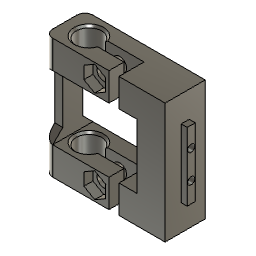
NAN dovetail rod mount - concept 2 v13 (Autodesk Fusion 360 design; units mm, degrees)
Autodesk Fusion 360 part; units mm, degrees
sketch "Sketch1" plane through (0, 0, 0) normal (0, 1, 0) x (1, 0, 0)
  line L0 (15, 15) -> (-15, 15)
  line L1 (-15, 15) -> (-15, -15)
  line L2 (-15, -15) -> (15, -15)
  line L3 (15, -15) -> (15, 15)
  line L4 (15, 15) -> (-15, -15) construction
  line L5 (-15, 15) -> (15, -15) construction
  dimension "d1" = 30
  dimension "d2" = 30
  constraint horizontal L0
  constraint perpendicular L0 L1
  constraint parallel L0 L2
  constraint parallel L1 L3
  constraint coincident L4 origin
  constraint coincident L5 origin
  measures "d1" distance of L1.end L2.end
  measures "d2" distance of L0.start L2.end
extrude "Extrude1" add sketch "Sketch1" along normal mid plane 10
sketch "Sketch2" plane through (0, 0, 15) normal (0, 0, 1) x (-1, 0, 0)
  line L0 (-15, 5) -> (-15, -5)
  line L1 (-15, -5) -> (15, -5)
  line L2 (15, -5) -> (15, 5)
  line L3 (15, 5) -> (-15, 5)
  point P0 (9, 0)
  dimension "d5" = 6
  measures "d5" distance of L2 P0
hole "Hole1" at (-9, 0, 15) direction (0, 0, -1) diameter 6.35 end through all
sketch "Sketch3" plane through (0, 0, 15) normal (0, 0, 1) x (-1, 0, 0)
  circle A0 centre (9, 0) radius 3.175
  line L0 (-15, 5) -> (-15, -5)
  line L1 (-15, -5) -> (15, -5)
  line L2 (15, -5) -> (15, 5)
  line L3 (15, 5) -> (-15, 5)
  line L4 (-3.5, -1.25) -> (11.5, -1.25)
  line L5 (11.5, -1.25) -> (11.5, 1.25)
  line L6 (11.5, 1.25) -> (-3.5, 1.25)
  line L7 (-3.5, 1.25) -> (-3.5, -1.25)
  line L8 (-3.5, -1.25) -> (11.5, 1.25) construction
  line L9 (11.5, -1.25) -> (-3.5, 1.25) construction
  line L10 (-3.5, 1.25) -> (-1, 1.25)
  line L11 (-1, 1.25) -> (-1, 5)
  line L12 (-3.5, 5) -> (-3.5, 1.25)
  point P0 (4, 0)
  dimension "d9" = 5
  dimension "d10" = 2.5
  dimension "d11" = 15
  dimension "d18" = 2.5
  constraint horizontal L4
  constraint perpendicular L4 L5
  constraint parallel L4 L6
  constraint parallel L5 L7
  constraint coincident L8 P0
  constraint coincident L9 P0
  constraint horizontal A0.centre P0
  constraint horizontal L10
  constraint vertical L11
  constraint vertical L12
  constraint coincident L3 L11.end
  constraint coincident L3 L12.start
  measures "d9" distance of A0.centre P0
  measures "d10" distance of L4.start L6.end
  measures "d11" distance of L5.end L6.end
  measures "d18" distance of L11 L12
extrude "Extrude2" cut sketch "Sketch3" against normal through all contours A0 L4 L6 L7 L10 | L3 L6 L10 L11 L12
sketch "Sketch4" plane through (0, 5, 0) normal (0, 1, 0) x (-1, 0, 0)
  line L0 (-15, 15) -> (-15, -15)
  line L1 (-15, -15) -> (15, -15)
  line L2 (15, -15) -> (15, 15)
  line L3 (15, 15) -> (-15, 15)
  line L4 (-1, -15) -> (6.0814, -15)
  line L5 (6.0814, -15) -> (6.0814, 15)
  line L6 (6.0814, 15) -> (-1, 15)
  line L7 (-1, 15) -> (-1, -15)
  point P0 (2.5407, 11.5)
  point P1 (2.5407, 15)
  dimension "d14" = 3.5
  constraint midpoint L6 P1
  constraint vertical P0 P1
  measures "d14" distance of P0 P1
hole "Hole2" at (-2.5407, 5, 11.5) direction (0, -1, 0) diameter 3.4 depth 10 tip angle 118
sketch "Sketch5" plane through (0, -5, 0) normal (0, -1, 0) x (1, 0, 0)
  circle A0 centre (-2.5407, 11.5) radius 1.7
  line L0 (1, -15) -> (1, 15)
  line L1 (1, 15) -> (-15, 15)
  line L2 (-15, 15) -> (-15, -15)
  line L3 (-15, -15) -> (1, -15)
  line L4 (0.1613, 9.94) -> (0.1613, 13.06)
  line L5 (0.1613, 13.06) -> (-2.5407, 14.62)
  line L6 (-2.5407, 14.62) -> (-5.2427, 13.06)
  line L7 (-5.2427, 13.06) -> (-5.2427, 9.94)
  line L8 (-5.2427, 9.94) -> (-2.5407, 8.38)
  line L9 (-2.5407, 8.38) -> (0.1613, 9.94)
  point P0 (-2.5407, 11.5)
  dimension "d19" = 3.12
  constraint coincident P0 A0.centre
  constraint vertical L5.end P0
  measures "d19" distance of L5.end P0
extrude "Extrude3" cut sketch "Sketch5" against normal blind 2.25 contours L4 L5 L6 L7 L8 L9
mirror "Mirror1" about plane through (0, 0, 0) normal (0, 0, 1) of "Hole2", "Extrude3"
sketch "Sketch6" plane through (0, 5, 0) normal (0, 1, 0) x (-1, 0, 0)
  circle A0 centre (2.5407, -11.5) radius 1.7
  circle A1 centre (2.5407, 11.5) radius 1.7
  line L0 (-15, 15) -> (-15, -15)
  line L1 (-15, -15) -> (15, -15)
  line L2 (15, -15) -> (15, 15)
  line L3 (15, 15) -> (-15, 15)
  line L4 (13, 8) -> (-8, 8)
  line L5 (-8, 8) -> (-8, -8)
  line L6 (-8, -8) -> (13, -8)
  line L7 (13, -8) -> (13, 8)
  dimension "d24" = 7
  dimension "d25" = 7
  dimension "d26" = 7
  dimension "d27" = 2
  constraint horizontal L4
  constraint vertical L5
  constraint horizontal L6
  constraint vertical L6.end L4.start
  measures "d24" distance of L0 L5
  measures "d25" distance of L3 L4
  measures "d26" distance of L1 L6
  measures "d27" distance of L2 L7
extrude "Extrude4" cut sketch "Sketch6" against normal through all contours L4 L5 L6 L7
sketch "Sketch7" plane through (15, 0, 0) normal (1, 0, 0) x (0, 1, 0)
  line L0 (-5, -15) -> (5, -15)
  line L1 (5, -15) -> (5, 15)
  line L2 (5, 15) -> (-5, 15)
  line L3 (-5, 15) -> (-5, -15)
  line L4 (1, -8.5) -> (-1, -8.5)
  line L5 (-1, -8.5) -> (-1, 8.5)
  line L6 (-1, 8.5) -> (1, 8.5)
  line L7 (1, 8.5) -> (1, -8.5)
  line L8 (1, -8.5) -> (-1, 8.5) construction
  line L9 (-1, -8.5) -> (1, 8.5) construction
  dimension "d29" = 2
  dimension "d30" = 17
  constraint horizontal L4
  constraint perpendicular L4 L5
  constraint parallel L4 L6
  constraint parallel L5 L7
  constraint coincident L8 origin
  constraint coincident L9 origin
  measures "d29" distance of L5.end L6.end
  measures "d30" distance of L4.start L6.end
extrude "Extrude5" add sketch "Sketch7" along normal blind 1.5 contours L4 L5 L6 L7
sketch "Sketch8" plane through (16.5, 0, 0) normal (1, 0, 0) x (0, 1, 0)
  line L0 (1, 8.5) -> (-1, 8.5)
  line L1 (-1, 8.5) -> (-1, -8.5)
  line L2 (-1, -8.5) -> (1, -8.5)
  line L3 (1, -8.5) -> (1, 8.5)
  point P0 (0, 3.5)
  point P1 (0, -3.5)
  dimension "d33" = 3.5
  dimension "d34" = 3.5
  constraint vertical P0 P1
  measures "d33" distance of origin P0
  measures "d34" distance of origin P1
hole "Hole3" at (16.5, 0, 3.5) at (16.5, 0, -3.5) direction (-1, 0, 0) diameter 1.8 depth 8.5 tip angle 180
sketch "Sketch9" plane through (-15, 0, 0) normal (-1, 0, 0) x (0, -1, 0)
  line L0 (5, 15) -> (-5, 15)
  line L1 (-5, 15) -> (-5, -15)
  line L2 (-5, -15) -> (5, -15)
  line L3 (5, -15) -> (5, 15)
  line L4 (-5, 8) -> (5, 8)
  line L5 (-5, 8) -> (-2.5, 5.5)
  line L6 (-2.5, 5.5) -> (-2.5, -5.5)
  line L7 (-5, -8) -> (5, -8)
  line L8 (-2.5, -5.5) -> (-5, -8)
  line L9 (-5, 8) -> (-5, -8)
  point P0 (-5, -8)
  dimension "d38" = 135
  dimension "d39" = 135
  dimension "d40" = 2.5
  constraint coincident L4.start L5.start
  constraint perpendicular L4 L6
  constraint coincident P0 L7.start
  measures "d38" angle of L6 L8
  measures "d39" angle of L5 L6
  measures "d40" distance of L6 L9
extrude "Extrude6" cut sketch "Sketch9" against normal up to surface (2 mm away) contours L1 L5 L6 L8 L9
chamfer "Chamfer1" distance 0.5 angle 45 4 edges at (-12.175, 0, -15) (-12.175, 0, -8) (-12.175, 0, 8) (-12.175, 0, 15)
mirror "Mirror2" about plane through (0, 0, 0) normal (0, 1, 0) of "Extrude6"
fillet "Fillet1" radius 2 1 edges at (-15, -5, 11.5)
fillet "Fillet1" radius 2 1 edges at (-15, 5, 11.5)
fillet "Fillet1" radius 2 2 edges at (-15, 5, -11.5) (-15, -5, -11.5)
